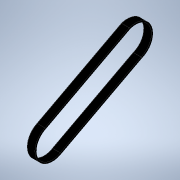
# Autodesk Inventor part: Adrian_Riemen
Saved by Autodesk Inventor 2021 (Build 250183000, 183)
## iProperties
Created: 2022-07-12
Part Number: Adrian_Riemen
Material: Generisch
Document SubType Name: Modeling
Designer: adria
Mass: 1.56139 g
Surface Area: 34.8422 cm^2
Volume: 1.56139 cm^3
Density: 1 g/cm^3
Appearance: Vorgabe
Author: adria
Autodesk Inventor part; units mm, degrees
ref_plane "YZ Plane" through (0, 0, 0) normal (1, 0, 0) x (0, 1, 0)
ref_plane "XZ Plane" through (0, 0, 0) normal (0, 1, 0) x (-1, 0, 0)
ref_plane "XY Plane" through (0, 0, 0) normal (0, 0, 1) x (1, 0, 0)
sketch "Skizze1" plane through (0, 0, 0) normal (1, 0, 0) x (0, 1, 0)
  circle A0 centre (0, 0) radius 13 construction
  circle A1 centre (34.5, -65.5) radius 13 construction
  line L0 (11.8104, 5.4728) -> (46.7538, -60.869)
  line L1 (-11.1936, -6.6438) -> (22.2462, -70.131)
  arc A2 (22.2462, -70.131) -> (46.7538, -60.869) centre (34.5, -65.5) ccw
  arc A3 (11.8104, 5.4728) -> (-11.1936, -6.6438) centre (0, 0) ccw
  dimension "d0" = 26
  dimension "d1" = 26
  dimension "d2" = 65.5
  dimension "d3" = 34.5
  constraints: 4 centre point, 4 end point, 4 point on circle, 4 tangent, 3 coincident
  measures "d0" diameter of A0
  measures "d1" diameter of A1
  measures "d2" vertical distance of A1.centre A0.centre
  measures "d3" horizontal distance of A0.centre A1.centre
sketch "Skizze2" plane through (0, 0, 0) normal (0, 0, 1) x (1, 0, 0)
  line L0 (0, -11.1936) -> (0, 22.2462) projected
  line L1 (-3, -13.0168) -> (3, -13.0168) construction
  line L2 (-3, -13.5168) -> (3, -13.5168)
  line L3 (3, -12.5168) -> (-3, -12.5168)
  arc A0 (-3, -12.5168) -> (-3, -13.5168) centre (-3, -13.0168) ccw
  arc A1 (3, -13.5168) -> (3, -12.5168) centre (3, -13.0168) ccw
  line L4 (0, -13.0168) -> (0, 11.8104) projected
  line L5 (0, 11.8104) -> (0, 46.7538) projected
  point P0 (0, 0)
  dimension "d4" = 1
  dimension "d5" = 7
  constraints: 8 end point, 4 point on circle, 4 tangent, 2 centre point, 1 horizontal, 1 midpoint, 1 parallel
  measures "d4" distance between parallel lines of L2 L3
sweep "Sweeping1" add profiles "Skizze2" path "Skizze1"
equation "\"d1\" = d0"
